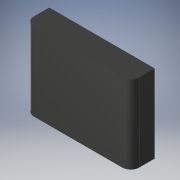
# Autodesk Inventor part: BatteryHolder
Saved by Autodesk Inventor 2018 (Build 220112000, 112)
## iProperties
Created: 2018-01-13
Part Number: BatteryHolder
Material: ABS Plastic
Document SubType Name: Modeling
Designer: Kyle-HP
Density: 1.06 g/cm^3
Appearance: Smooth - Black
Author: Kyle-HP
Autodesk Inventor part; units mm, degrees
ref_plane "YZ Plane" through (0, 0, 0) normal (1, 0, 0) x (0, 1, 0)
ref_plane "XZ Plane" through (0, 0, 0) normal (0, 1, 0) x (-1, 0, 0)
ref_plane "XY Plane" through (0, 0, 0) normal (0, 0, 1) x (1, 0, 0)
sketch "Sketch1" plane through (0, 0, 0) normal (0, 0, 1) x (1, 0, 0)
  line L0 (0, 0) -> (78.74, 0)
  line L1 (78.74, 0) -> (78.74, -58.42)
  line L2 (78.74, -58.42) -> (0, -58.42)
  line L3 (0, -58.42) -> (0, 0)
  dimension "d0" = 78.74
  dimension "d1" = 58.42
  constraints: 8 end point, 2 parallel, 1 horizontal, 1 perpendicular
  measures "d0" distance of L0.start L0.end
  measures "d1" distance of L2.end L0.start
extrude "Extrusion1" add sketch "Sketch1" along normal blind 17.78
fillet "Fillet1" radius 6.35 2 edges at (78.74, -29.21, 17.78) (0, -29.21, 17.78)
body "Solid1"
